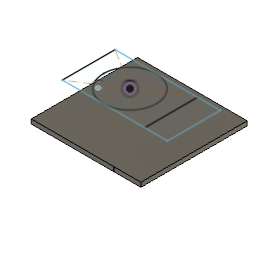
bearing fit arm (Autodesk Fusion 360 design; units mm, degrees)
part number: 2026-01-16-14-08-22-554
Autodesk Fusion 360 part; units mm, degrees
sketch "Sketch1" plane through (0, 0, 0) normal (0, 0, 1) x (1, 0, 0)
  circle A0 centre (0, 0) radius 10.1
  dimension "d1" = 20.2
  constraint coincident A0.centre origin
  measures "d1" diameter of A0
extrude "Extrude1" add sketch "Sketch1" along normal blind 13.95
sketch "Sketch2" plane through (0, 0, 13.95) normal (0, 0, 1) x (-1, 0, 0)
  circle A0 centre (0, 0) radius 10.1
  circle A1 centre (0, 0) radius 17.5
  line L0 (-27.5, -17.6099) -> (27.5, -17.6099)
  line L1 (27.5, -17.6099) -> (27.5, 17.6099)
  line L2 (27.5, 17.6099) -> (-27.5, 17.6099)
  line L3 (-27.5, 17.6099) -> (-27.5, -17.6099)
  line L4 (-27.5, -17.6099) -> (27.5, 17.6099) construction
  line L5 (27.5, -17.6099) -> (-27.5, 17.6099) construction
  line L6 (-27.5, -17.6099) -> (-42.678, -17.6099)
  line L7 (-42.678, -17.6099) -> (-42.678, 17.6539)
  line L8 (-42.678, 17.6539) -> (-27.5, 17.6539)
  line L9 (-27.5, 17.6539) -> (-27.5, -17.6099)
  dimension "d4" = 35
  dimension "d7" = 55
  constraint coincident A0.centre A1.centre
  constraint horizontal L0
  constraint perpendicular L0 L1
  constraint parallel L0 L2
  constraint parallel L1 L3
  constraint coincident L4 A0.centre
  constraint coincident L5 A0.centre
  constraint horizontal L6
  constraint vertical L7
  constraint horizontal L8
  constraint vertical L9
  measures "d4" diameter of A1
  measures "d7" distance of L1.end L2.end
extrude "Extrude2" add sketch "Sketch2" along normal blind 2 contours A0 | A1
extrude "Extrude3" add sketch "Sketch2" along normal blind 2 contours L0 L1 L2 L3 L9
sketch "Sketch3" plane through (0, 0, 13.95) normal (0, 0, 1) x (-1, 0, 0)
  circle A0 centre (11.0543, 10.2607) radius 1.5
  dimension "d10" = 3
  measures "d10" diameter of A0
extrude "Extrude4" add sketch "Sketch2" along normal blind 2 contours L3 L6 L7 L8 L9
sketch "Sketch5" plane through (0, -17.6099, 0) normal (0, -1, 0) x (1, 0, 0)
  line L0 (-27.5, 13.95) -> (27.5, 13.95)
  line L1 (27.5, 13.95) -> (27.5, 15.95)
  line L2 (27.5, 15.95) -> (-27.5, 15.95)
  line L3 (-27.5, 15.95) -> (-27.5, 13.95)
  line L4 (-27.5, 15.95) -> (42.6781, 15.95)
  line L5 (42.6781, 15.95) -> (42.6781, 13.95)
  line L6 (42.6781, 13.95) -> (-27.5, 13.95)
  line L7 (-27.5, 13.95) -> (-27.5, 15.95)
  constraint horizontal L4
  constraint vertical L5
  constraint horizontal L6
  constraint vertical L7
  constraint coincident L2.end L3.start
extrude "Extrude5" add sketch "Sketch5" along normal blind 35.8
sketch "Sketch6" plane through (42.678, 0, 0) normal (1, 0, 0) x (0, 1, 0)
  line L0 (-17.6099, 15.95) -> (-17.6099, 13.95)
  line L1 (-17.6099, 13.95) -> (17.6099, 13.95)
  line L2 (17.6099, 13.95) -> (17.6099, 15.95)
  line L3 (17.6099, 15.95) -> (-17.6099, 15.95)
  line L4 (17.6099, 15.95) -> (-53.4009, 15.95)
  line L5 (-53.4009, 15.95) -> (-53.4009, 13.9526)
  line L6 (-53.4009, 13.9526) -> (17.6099, 13.9526)
  line L7 (17.6099, 13.9526) -> (17.6099, 15.95)
  constraint horizontal L4
  constraint vertical L5
  constraint horizontal L6
  constraint vertical L7
  constraint coincident L2.end L3.start
extrude "Extrude6" add sketch "Sketch6" along normal blind 18 contours L0 L2 L3 L4 L6 L7 | L0 L4 L5 L6
sketch "Sketch7" plane through (-27.5, 0, 0) normal (-1, 0, 0) x (0, -1, 0)
  line L0 (-17.6099, 13.95) -> (53.4099, 13.95)
  line L1 (53.4099, 13.95) -> (53.4099, 15.95)
  line L2 (53.4099, 15.95) -> (-17.6099, 15.95)
  line L3 (-17.6099, 15.95) -> (-17.6099, 13.95)
  line L4 (-17.6099, 15.95) -> (53.4099, 15.95)
  line L5 (53.4099, 15.95) -> (53.4099, 13.95)
  line L6 (53.4099, 13.95) -> (-17.6099, 13.95)
  line L7 (-17.6099, 13.95) -> (-17.6099, 15.95)
  constraint horizontal L4
  constraint vertical L5
  constraint horizontal L6
  constraint vertical L7
  constraint coincident L0.end L1.start
  constraint coincident L2.end L3.start
extrude "Extrude7" cut sketch "Sketch7" against normal blind 15
sketch "Sketch8" plane through (0, 0, 13.95) normal (0, 0, 1) x (-1, 0, 0)
  circle A0 centre (0, 0) radius 12.0416
  constraint coincident A0.centre origin
extrude "Extrude8" add sketch "Sketch8" against normal blind 2
extrude "Extrude9" add 1 faces at (30.2854, -6.0604, 15.95) along direction (0, 0, 1) blind 1
